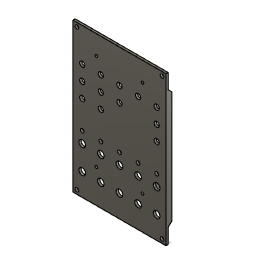
CB55 - Faceplate (Autodesk Fusion 360 design; units mm, degrees)
Autodesk Fusion 360 part; units mm, degrees
note: some values were not read from the file. Set by a fixed rule: which sketch regions a step uses.
sketch "Sketch1" plane through (0, 0, 0) normal (0, 0, 1) x (1, 0, 0)
  line L0 (5, 5) -> (130, 5)
  line L1 (130, 5) -> (130, 205)
  line L2 (130, 205) -> (5, 205)
  line L3 (5, 205) -> (5, 5)
  line L4 (5, 5) -> (31.5, 5)
  line L5 (31.5, 5) -> (31.5, 45)
  line L6 (31.5, 45) -> (103.5, 45)
  line L7 (103.5, 45) -> (103.5, 184)
  line L8 (103.5, 184) -> (31.5, 184)
  line L9 (31.5, 184) -> (31.5, 45)
  line L10 (31.5, 45) -> (36.5, 45)
  line L11 (36.5, 45) -> (36.5, 50)
  circle A0 centre (36.5, 50) radius 1.75
  line L12 (103.5, 45) -> (98.5, 45)
  line L13 (98.5, 45) -> (98.5, 50)
  circle A1 centre (98.5, 50) radius 1.75
  line L14 (31.5, 184) -> (36.5, 184)
  line L15 (36.5, 184) -> (36.5, 179)
  circle A2 centre (36.5, 179) radius 1.75
  line L16 (103.5, 184) -> (103.5, 179)
  line L17 (103.5, 179) -> (98.5, 179)
  circle A3 centre (98.5, 179) radius 1.75
  dimension "d1" = 125
  dimension "d2" = 200
  dimension "d58" = 26.5
  dimension "d59" = 40
  dimension "d60" = 72
  dimension "d61" = 139
  dimension "d62" = 5
  dimension "d63" = 5
  dimension "d64" = 3.5
  dimension "d65" = 5
  dimension "d66" = 5
  dimension "d67" = 3.5
  dimension "d68" = 5
  dimension "d69" = 5
  dimension "d70" = 3.5
  dimension "d71" = 5
  dimension "d72" = 5
  dimension "d73" = 3.5
  constraint horizontal L0
  constraint vertical L1
  constraint horizontal L2
  constraint vertical L3
  constraint perpendicular L3 L4
  constraint perpendicular L0 L5
  constraint horizontal L6
  constraint vertical L7
  constraint horizontal L8
  constraint vertical L9
  constraint perpendicular L9 L10
  constraint perpendicular L10 L11
  constraint coincident L11.end A0.centre
  constraint perpendicular L7 L12
  constraint perpendicular L12 L13
  constraint coincident L13.end A1.centre
  constraint perpendicular L9 L14
  constraint perpendicular L14 L15
  constraint coincident L15.end A2.centre
  constraint perpendicular L8 L16
  constraint perpendicular L16 L17
  constraint coincident L17.end A3.centre
  measures "d1" distance of L0.start L0.end
  measures "d2" distance of L0.start L2.end
  measures "d58" distance of L0.start L4.end
  measures "d59" distance of L4.end L5.end
  measures "d60" distance of L5.end L6.end
  measures "d61" distance of L5.end L8.end
  measures "d62" distance of L5.end L10.end
  measures "d63" distance of L10.end L11.end
  measures "d64" diameter of A0
  measures "d65" distance of L6.end L12.end
  measures "d66" distance of L12.end L13.end
  measures "d67" diameter of A1
  measures "d68" distance of L8.end L14.end
  measures "d69" distance of L14.end L15.end
  measures "d70" diameter of A2
  measures "d71" distance of L7.end L16.end
  measures "d72" distance of L16.end L17.end
  measures "d73" diameter of A3
extrude "Extrude1" add sketch "Sketch1" along normal blind 3 contours L0 L1 L2 L3 L4 | L6 L7 L8 L9 L10 L12 L14 L16
sketch "Sketch2" plane through (0, 0, 0) normal (0, 0, -1) x (-1, 0, 0)
  line L0 (-5, 5) -> (-5, 205)
  line L1 (-5, 205) -> (-130, 205)
  line L2 (-130, 205) -> (-130, 5)
  line L3 (-130, 5) -> (-5, 5)
  line L4 (-130, 205) -> (-130, 185)
  line L5 (-130, 5) -> (-130, 25)
  line L6 (-130, 185) -> (-127, 185)
  line L7 (-127, 185) -> (-127, 25)
  line L8 (-127, 25) -> (-130, 25)
  line L9 (-130, 25) -> (-130, 185)
  line L10 (-8, 185) -> (-8, 25)
  line L11 (-5, 25) -> (-5, 185)
  line L12 (-5, 185) -> (-8, 185)
  line L13 (-5, 205) -> (-5, 185)
  line L14 (-8, 25) -> (-5, 25)
  line L15 (-5, 5) -> (-5, 25)
  line L16 (-5, 205) -> (-10.3033, 199.6967)
  line L17 (-5, 205) -> (-10, 205) construction
  line L18 (-5, 5) -> (-10.3033, 10.3033)
  line L19 (-5, 5) -> (-10, 5) construction
  circle A0 centre (-10.3033, 10.3033) radius 2.5
  circle A1 centre (-10.3033, 199.6967) radius 2.5
  circle A2 centre (-124.6967, 199.6967) radius 2.5
  line L20 (-130, 205) -> (-124.6967, 199.6967)
  line L21 (-130, 5) -> (-124.6967, 10.3033)
  circle A3 centre (-124.6967, 10.3033) radius 2.5
  line L22 (-67.5, 205) -> (-130, 205)
  line L23 (-67.5, 205) -> (-5, 205)
  line L24 (-30, 205) -> (-30, 5)
  line L25 (-30, 205) -> (-5, 205)
  line L26 (-5, 185) -> (-5, 205)
  line L27 (-5, 185) -> (-8, 185)
  line L28 (-8, 185) -> (-8, 25)
  line L29 (-8, 25) -> (-5, 25)
  line L30 (-5, 25) -> (-5, 5)
  line L31 (-5, 5) -> (-30, 5)
  line L32 (-30, 205) -> (-67.5, 205)
  line L33 (-67.5, 5) -> (-36.25, 5)
  line L34 (-67.5, 5) -> (-98.75, 5)
  line L35 (-67.5, 205) -> (-130, 205)
  line L36 (-130, 205) -> (-130, 185)
  line L37 (-127, 185) -> (-127, 25)
  line L38 (-130, 5) -> (-130, 25)
  line L39 (-130, 5) -> (-98.75, 5)
  line L40 (-130, 185) -> (-127, 185)
  line L41 (-30, 205) -> (-55, 205)
  line L42 (-55, 205) -> (-55, 5)
  line L43 (-55, 5) -> (-30, 5)
  line L44 (-30, 5) -> (-30, 205)
  line L45 (-55, 205) -> (-80, 205)
  line L46 (-80, 205) -> (-80, 5)
  line L47 (-80, 5) -> (-55, 5)
  line L48 (-55, 5) -> (-55, 205)
  line L49 (-80, 205) -> (-105, 205)
  line L50 (-105, 205) -> (-105, 5)
  line L51 (-105, 5) -> (-80, 5)
  line L52 (-80, 5) -> (-80, 205)
  circle A4 centre (-98.5, 50) radius 1.75
  circle A5 centre (-98.5, 179) radius 1.75
  circle A6 centre (-36.5, 50) radius 1.75
  circle A7 centre (-36.5, 179) radius 1.75
  dimension "d6" = 20
  dimension "d7" = 3
  dimension "d8" = 45
  dimension "d9" = 7.5
  dimension "d10" = 45
  dimension "d11" = 7.5
  dimension "d12" = 5
  dimension "d13" = 5
  dimension "d20" = 160
  dimension "d21" = 20
  dimension "d23" = 200
  dimension "d38" = 25
  dimension "d39" = 25
  dimension "d40" = 25
  dimension "d41" = 25
  constraint coincident L1.end L2.start
  constraint coincident L2 L4.end
  constraint perpendicular L1 L4
  constraint coincident L2.end L3.start
  constraint perpendicular L3 L5
  constraint horizontal L6
  constraint vertical L7
  constraint horizontal L8
  constraint vertical L9
  constraint midpoint L3 L33.start
  constraint horizontal L17
  constraint horizontal L19
  constraint coincident L18.end A0.centre
  constraint coincident L16.end A1.centre
  constraint coincident L0.end L1.start
  constraint perpendicular L23 L24
  constraint coincident L0.start L3.end
  constraint horizontal L32
  constraint horizontal L33
  constraint horizontal L41
  constraint vertical L42
  constraint horizontal L43
  constraint vertical L44
  constraint horizontal L45
  constraint vertical L46
  constraint horizontal L47
  constraint vertical L48
  constraint horizontal L49
  constraint vertical L50
  constraint horizontal L51
  constraint vertical L52
  measures "d6" distance of L2.end L5.end
  measures "d7" distance of L4.end L6.end
  measures "d8" angle of L16 L17
  measures "d9" distance of L0.end L16.end
  measures "d10" angle of L18 L19
  measures "d11" distance of L0.start L18.end
  measures "d12" diameter of A0
  measures "d13" diameter of A1
  measures "d20" distance of L6.end L7.end
  measures "d21" distance of L1.end L4.end
  measures "d23" distance of L24.start L24.end
  measures "d38" distance of L24.end L0.start
  measures "d39" distance of L24.start L41.end
  measures "d40" distance of L41.end L45.end
  measures "d41" distance of L45.end L49.end
extrude "Extrude2" cut sketch "Sketch2" against normal blind 3 contours A1
extrude "Extrude3" cut sketch "Sketch2" against normal blind 3 contours A0 | A2 | A3
extrude "Extrude4" add sketch "Sketch2" along normal blind 5 contours L0 L10 L11 L12 L14 L27 L28 L29 | L2 L6 L7 L8 L9 L37 L40
sketch "Sketch3" plane through (0, 0, 3) normal (0, 0, 1) x (1, 0, 0)
  circle A0 centre (124.6967, 199.6967) radius 2.5
  circle A1 centre (124.6967, 10.3033) radius 2.5
  circle A2 centre (10.3033, 10.3033) radius 2.5
  circle A3 centre (10.3033, 199.6967) radius 2.5
  line L0 (5, 205) -> (5, 5)
  line L1 (5, 5) -> (130, 5)
  line L2 (130, 5) -> (130, 205)
  line L3 (130, 205) -> (5, 205)
  line L4 (5, 5) -> (5, 35)
  line L5 (5, 5) -> (30, 5)
  line L6 (5, 35) -> (17.5, 35)
  circle A4 centre (17.5, 35) radius 4.5
  line L7 (17.5, 35) -> (17.5, 67.5)
  circle A5 centre (17.5, 67.5) radius 4.5
  line L8 (17.5, 67.5) -> (17.5, 120)
  circle A6 centre (17.5, 120) radius 3.5
  line L9 (17.5, 120) -> (17.5, 140)
  circle A7 centre (17.5, 140) radius 3.5
  line L10 (17.5, 140) -> (17.5, 160)
  circle A8 centre (17.5, 160) radius 3.5
  line L11 (130, 5) -> (98.75, 5)
  line L12 (30, 5) -> (30, 205)
  circle A9 centre (42.5, 160) radius 3.5
  circle A10 centre (42.5, 140) radius 3.5
  circle A11 centre (42.5, 67.5) radius 4.5
  circle A12 centre (42.5, 120) radius 3.5
  circle A13 centre (42.5, 35) radius 4.5
  line L13 (55, 205) -> (55, 5)
  circle A14 centre (67.5, 160) radius 3.5
  circle A15 centre (67.5, 140) radius 3.5
  circle A16 centre (67.5, 67.5) radius 4.5
  circle A17 centre (67.5, 35) radius 4.5
  line L14 (80, 5) -> (80, 205)
  circle A18 centre (92.5, 160) radius 3.5
  circle A19 centre (92.5, 67.5) radius 4.5
  circle A20 centre (92.5, 35) radius 4.5
  line L15 (80, 205) -> (80, 5)
  circle A21 centre (117.5, 160) radius 3.5
  circle A22 centre (117.5, 140) radius 3.5
  circle A23 centre (117.5, 120) radius 3.5
  circle A24 centre (117.5, 67.5) radius 4.5
  circle A25 centre (117.5, 35) radius 4.5
  line L16 (17.5, 67.5) -> (17.5, 82.5)
  circle A26 centre (17.5, 82.5) radius 2.5
  circle A27 centre (42.5, 82.5) radius 2.5
  circle A28 centre (67.5, 82.5) radius 2.5
  circle A29 centre (92.5, 82.5) radius 2.5
  line L17 (105, 205) -> (105, 5)
  circle A30 centre (117.5, 82.5) radius 2.5
  circle A31 centre (98.5, 50) radius 1.75
  circle A32 centre (98.5, 179) radius 1.75
  circle A33 centre (36.5, 50) radius 1.75
  circle A34 centre (36.5, 179) radius 1.75
  dimension "d24" = 30
  dimension "d25" = 31.25
  dimension "d26" = 12.5
  dimension "d27" = 9
  dimension "d28" = 32.5
  dimension "d29" = 9
  dimension "d30" = 52.5
  dimension "d31" = 7
  dimension "d32" = 20
  dimension "d33" = 7
  dimension "d34" = 20
  dimension "d35" = 7
  dimension "d36" = 31.25
  dimension "d42" = 15
  dimension "d43" = 5
  constraint coincident L0.end L1.start
  constraint perpendicular L1 L4
  constraint perpendicular L0 L6
  constraint coincident L6.end A4.centre
  constraint perpendicular L6 L7
  constraint coincident L7.end A5.centre
  constraint parallel L7 L8
  constraint coincident L8.end A6.centre
  constraint parallel L8 L9
  constraint coincident L9.end A7.centre
  constraint parallel L9 L10
  constraint coincident L10.end A8.centre
  constraint coincident L1.end L2.start
  constraint perpendicular L2 L11
  constraint symmetric A4 L12 A13
  constraint symmetric A5 L12 A11
  constraint symmetric A6 L12 A12
  constraint symmetric A7 L12 A10
  constraint symmetric A8 L12 A9
  constraint symmetric A9 L13 A14
  constraint symmetric A10 L13 A15
  constraint symmetric A11 L13 A16
  constraint symmetric A13 L13 A17
  constraint symmetric A14 L14 A18
  constraint symmetric A16 L14 A19
  constraint symmetric A17 L14 A20
  constraint symmetric A9 L15 A21
  constraint symmetric A10 L15 A22
  constraint symmetric A11 L15 A24
  constraint symmetric A12 L15 A23
  constraint symmetric A13 L15 A25
  constraint parallel L8 L16
  constraint coincident L16.end A26.centre
  constraint symmetric L12 A26 A27
  constraint symmetric L13 A27 A28
  constraint symmetric L15 A28 A29
  constraint symmetric A29 L17 A30
  measures "d24" distance of L0.end L4.end
  measures "d26" distance of L4.end L6.end
  measures "d27" diameter of A4
  measures "d28" distance of L6.end L7.end
  measures "d29" diameter of A5
  measures "d30" distance of L7.end L8.end
  measures "d31" diameter of A6
  measures "d32" distance of L8.end L9.end
  measures "d33" diameter of A7
  measures "d34" distance of L9.end L10.end
  measures "d35" diameter of A8
  measures "d36" distance of L1.end L11.end
  measures "d42" distance of L7.end L16.end
  measures "d43" diameter of A26
extrude "Extrude5" cut sketch "Sketch3" against normal blind 3 contours L6 A4 L7 | L6 A4 L7 | L7 A5 L8 L16 | L7 A5 L8 L16 | L8 L16 A26 | L8 L16 A26 | L8 A6 L9 | L8 A6 L9 | L9 A7 L10 | L9 A7 L10 | A8 | A9 | A10 | A11 | A12 | A13 | A14 | A15 | A16 | A17 | A18 | A19 | A20 | A21 | A22 | A23 | A24 | A25 | A27 | A28 | A29 | A30
sketch "Sketch4" plane through (0, 0, 3) normal (0, 0, 1) x (1, 0, 0)
  circle A0 centre (117.5, 82.5) radius 2.5
  circle A1 centre (42.5, 160) radius 3.5
  circle A2 centre (92.5, 67.5) radius 4.5
  circle A3 centre (67.5, 82.5) radius 2.5
  circle A4 centre (42.5, 82.5) radius 2.5
  circle A5 centre (17.5, 67.5) radius 4.5
  circle A6 centre (17.5, 160) radius 3.5
  circle A7 centre (17.5, 82.5) radius 2.5
  circle A8 centre (42.5, 67.5) radius 4.5
  circle A9 centre (67.5, 140) radius 3.5
  circle A10 centre (92.5, 35) radius 4.5
  circle A11 centre (67.5, 160) radius 3.5
  circle A12 centre (117.5, 120) radius 3.5
  circle A13 centre (117.5, 67.5) radius 4.5
  circle A14 centre (117.5, 160) radius 3.5
  circle A15 centre (92.5, 82.5) radius 2.5
  circle A16 centre (67.5, 67.5) radius 4.5
  circle A17 centre (42.5, 120) radius 3.5
  circle A18 centre (17.5, 35) radius 4.5
  circle A19 centre (17.5, 140) radius 3.5
  circle A20 centre (17.5, 120) radius 3.5
  circle A21 centre (42.5, 35) radius 4.5
  circle A22 centre (42.5, 140) radius 3.5
  circle A23 centre (67.5, 35) radius 4.5
  circle A24 centre (92.5, 160) radius 3.5
  circle A25 centre (117.5, 140) radius 3.5
  circle A26 centre (117.5, 35) radius 4.5
  circle A27 centre (124.6967, 199.6967) radius 2.5
  circle A28 centre (124.6967, 10.3033) radius 2.5
  circle A29 centre (10.3033, 10.3033) radius 2.5
  circle A30 centre (10.3033, 199.6967) radius 2.5
  line L0 (5, 205) -> (5, 5)
  line L1 (5, 5) -> (130, 5)
  line L2 (130, 5) -> (130, 205)
  line L3 (130, 205) -> (5, 205)
  line L4 (5, 205) -> (17.5, 205)
  line L5 (17.5, 205) -> (17.5, 5)
  line L6 (17.5, 205) -> (42.5, 205)
  line L7 (42.5, 205) -> (42.5, 5)
  line L8 (42.5, 5) -> (17.5, 5)
  line L9 (17.5, 5) -> (17.5, 205)
  line L10 (42.5, 205) -> (67.5, 205)
  line L11 (67.5, 205) -> (67.5, 5)
  line L12 (67.5, 5) -> (42.5, 5)
  line L13 (42.5, 5) -> (42.5, 205)
  line L14 (67.5, 205) -> (92.5, 205)
  line L15 (92.5, 205) -> (92.5, 5)
  line L16 (92.5, 5) -> (67.5, 5)
  line L17 (67.5, 5) -> (67.5, 205)
  line L18 (92.5, 205) -> (117.5, 205)
  line L19 (117.5, 205) -> (117.5, 5)
  line L20 (117.5, 5) -> (92.5, 5)
  line L21 (92.5, 5) -> (92.5, 205)
  line L22 (5, 205) -> (5, 185)
  line L23 (5, 185) -> (130, 185)
  circle A31 centre (98.5, 50) radius 1.75
  circle A32 centre (98.5, 179) radius 1.75
  circle A33 centre (36.5, 50) radius 1.75
  circle A34 centre (36.5, 179) radius 1.75
  dimension "d47" = 12.5
  dimension "d49" = 25
  dimension "d50" = 200
  dimension "d51" = 25
  dimension "d52" = 25
  dimension "d53" = 200
  dimension "d54" = 25
  dimension "d56" = 20
  dimension "d57" = 125
  constraint coincident L0.start L3.end
  constraint perpendicular L0 L4
  constraint vertical L5
  constraint horizontal L6
  constraint vertical L7
  constraint horizontal L8
  constraint vertical L9
  constraint horizontal L10
  constraint vertical L11
  constraint horizontal L12
  constraint vertical L13
  constraint horizontal L14
  constraint vertical L15
  constraint horizontal L16
  constraint vertical L17
  constraint horizontal L18
  constraint vertical L19
  constraint horizontal L20
  constraint vertical L21
  constraint coincident L0 L22.end
  constraint perpendicular L2 L23
  measures "d47" distance of L0.start L4.end
  measures "d49" distance of L4.end L6.end
  measures "d50" distance of L4.end L5.end
  measures "d51" distance of L6.end L10.end
  measures "d52" distance of L10.end L14.end
  measures "d53" distance of L10.end L11.end
  measures "d54" distance of L14.end L18.end
  measures "d56" distance of L0.start L22.end
  measures "d57" distance of L22.end L23.end
sketch "Sketch5" plane through (0, 0, 3) normal (0, 0, 1) x (1, 0, 0)
chamfer "Chamfer1" distance 5 angle 45 4 edges at (6.5, 185, -5) (6.5, 25, -5) (128.5, 25, -5) (128.5, 185, -5)
sketch "Sketch6" plane through (0, 0, 0) normal (0, 0, 1) x (1, 0, 0)
  circle A0 centre (98.5, 179) radius 3.5
  circle A1 centre (98.5, 50) radius 3.5
  circle A2 centre (98.5, 50) radius 1.75
  circle A3 centre (98.5, 179) radius 1.75
  line L0 (67.5, 205) -> (67.5, 5)
  circle A4 centre (36.5, 179) radius 3.5
  circle A5 centre (36.5, 179) radius 1.75
  circle A6 centre (36.5, 50) radius 3.5
  circle A7 centre (36.5, 50) radius 1.75
  dimension "d75" = 7
  dimension "d76" = 7
  dimension "d77" = 3.5
  dimension "d78" = 3.5
  constraint concentric A1 A2
  constraint concentric A0 A3
  constraint symmetric A0 L0 A4
  constraint symmetric A1 L0 A6
  constraint symmetric A2 L0 A7
  constraint symmetric A3 L0 A5
  measures "d75" diameter of A0
  measures "d76" diameter of A1
  measures "d77" diameter of A2
  measures "d78" diameter of A3
extrude "Extrude6" add sketch "Sketch6" against normal blind 20
